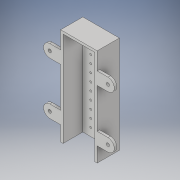
# Autodesk Inventor part: thermometerCover
Saved by Autodesk Inventor 2019.1 (Build 231200000, 200)
## iProperties
Created: 2018-08-04
Part Number: thermometerCover
Material: Generic
Document SubType Name: Modeling
Designer: steele
Density: 1 g/cm^3
Appearance: Default
Author: steele
Autodesk Inventor part; units mm, degrees
ref_plane "YZ Plane" through (0, 0, 0) normal (1, 0, 0) x (0, 1, 0)
ref_plane "XZ Plane" through (0, 0, 0) normal (0, 1, 0) x (-1, 0, 0)
ref_plane "XY Plane" through (0, 0, 0) normal (0, 0, 1) x (1, 0, 0)
sketch "Sketch1" plane through (0, 0, 0) normal (0, 0, 1) x (1, 0, 0)
  line L0 (25.4, -76.2) -> (25.4, 76.2)
  line L1 (25.4, 76.2) -> (-25.4, 76.2)
  line L2 (-25.4, 76.2) -> (-25.4, -76.2)
  line L3 (-25.4, -76.2) -> (25.4, 76.2) construction
  line L4 (25.4, -76.2) -> (-25.4, 76.2) construction
  line L5 (29.3687, -76.2) -> (29.3687, 80.1688)
  line L6 (29.3687, 80.1688) -> (-29.3687, 80.1688)
  line L7 (-29.3687, 80.1688) -> (-29.3687, -76.2)
  line L8 (-29.3687, -80.1688) -> (29.3687, 80.1688) construction
  line L9 (29.3687, -80.1688) -> (-29.3687, 80.1688) construction
  line L10 (-25.4, -76.2) -> (-29.3687, -76.2)
  line L11 (25.4, -76.2) -> (29.3687, -76.2)
  point P0 (0, 0)
  dimension "d2" = 3.9688
  dimension "d3" = 3.9688
  dimension "d5" = 50.8
  dimension "d6" = 152.4
  constraints: 24 end point, 4 midpoint, 2 parallel, 1 point on line
  measures "d2" distance between parallel lines of L5 L0
  measures "d3" distance between parallel lines of L6 L1
  measures "d5" distance between parallel lines of L0 L2
  measures "d6" distance of L0.start L0.end
extrude "Extrusion1" add sketch "Sketch1" along normal blind 31.75
sketch "Sketch2" plane through (0, 0, 0) normal (0, 0, -1) x (-1, 0, 0)
  line L0 (-29.3687, -76.2) -> (-29.3687, 80.1688) projected
  line L1 (29.3687, 80.1688) -> (29.3687, -76.2) projected
  line L2 (-29.3687, 80.1688) -> (29.3687, 80.1688)
  line L3 (29.3687, 80.1688) -> (29.3687, -76.2)
  line L4 (29.3687, -76.2) -> (-29.3687, -76.2)
  line L5 (-29.3687, -76.2) -> (-29.3687, 80.1688)
  point P0 (0, 0)
  constraints: 8 end point, 2 parallel, 1 horizontal, 1 perpendicular
extrude "Extrusion2" add sketch "Sketch2" along normal blind 3.9688
sketch "Sketch5" plane through (0, 0, 31.75) normal (0, 0, 1) x (1, 0, 0)
  line L0 (-29.3687, 80.1688) -> (-29.3687, -76.2)
  line L1 (-29.3687, 42.0688) -> (-46.7574, 42.0688) construction
  line L2 (-29.3687, 31.9088) -> (-46.7574, 31.9088)
  line L3 (-46.7574, 52.2287) -> (-29.3687, 52.2288)
  arc A0 (-46.7574, 52.2287) -> (-46.7574, 31.9088) centre (-46.7574, 42.0688) ccw
  line L4 (29.3687, 80.1688) -> (-29.3687, 80.1688)
  circle A1 centre (-46.7574, 42.0688) radius 2.54
  point P0 (0, 0)
  dimension "d18" = 10.16
  dimension "d21" = 5.08
  constraints: 8 end point, 2 centre point, 2 point on circle, 2 tangent, 1 coincident, 1 parallel, 1 perpendicular, 1 point on line
  measures "d18" radius of A0
  measures "d21" diameter of A1
extrude "Extrusion4" add sketch "Sketch5" against normal blind 3.9688
mirror "Mirror1" about plane through (0, 0, 0) normal (1, 0, 0) of "Extrusion4"
mirror "Mirror2" about plane through (0, 0, 0) normal (0, 1, 0) of "Extrusion4", "Mirror1"
sketch "Sketch6" plane through (0, 0, 0) normal (0, 0, 1) x (1, 0, 0)
  circle A0 centre (-12.7, -63.5) radius 1.5875
  line L0 (-25.4, -76.2) -> (-25.4, 76.2) projected
  line L1 (-25.4, -76.2) -> (25.4, -76.2) construction
  line L2 (-12.7, -63.5) -> (-12.7, 76.2) construction
  line L3 (-25.4, 76.2) -> (25.4, 76.2) construction
  line L4 (-12.7, -63.5) -> (25.4, -63.5) construction
  circle A1 centre (-12.7, -50.8) radius 1.5875
  circle A2 centre (-12.7, -38.1) radius 1.5875
  circle A3 centre (-12.7, -25.4) radius 1.5875
  circle A4 centre (-12.7, -12.7) radius 1.5875
  circle A5 centre (-12.7, 0) radius 1.5875
  circle A6 centre (-12.7, 12.7) radius 1.5875
  circle A7 centre (-12.7, 25.4) radius 1.5875
  circle A8 centre (-12.7, 38.1) radius 1.5875
  circle A9 centre (-12.7, 50.8) radius 1.5875
  circle A10 centre (-12.7, 63.5) radius 1.5875
  circle A11 centre (0, -63.5) radius 1.5875
  circle A12 centre (0, -50.8) radius 1.5875
  circle A13 centre (0, -38.1) radius 1.5875
  circle A14 centre (0, -25.4) radius 1.5875
  circle A15 centre (0, -12.7) radius 1.5875
  circle A16 centre (0, 0) radius 1.5875
  circle A17 centre (0, 12.7) radius 1.5875
  circle A18 centre (0, 25.4) radius 1.5875
  circle A19 centre (0, 38.1) radius 1.5875
  circle A20 centre (0, 50.8) radius 1.5875
  circle A21 centre (0, 63.5) radius 1.5875
  circle A22 centre (12.7, -63.5) radius 1.5875
  circle A23 centre (12.7, -50.8) radius 1.5875
  circle A24 centre (12.7, -38.1) radius 1.5875
  circle A25 centre (12.7, -25.4) radius 1.5875
  circle A26 centre (12.7, -12.7) radius 1.5875
  circle A27 centre (12.7, 0) radius 1.5875
  circle A28 centre (12.7, 12.7) radius 1.5875
  circle A29 centre (12.7, 25.4) radius 1.5875
  circle A30 centre (12.7, 38.1) radius 1.5875
  circle A31 centre (12.7, 50.8) radius 1.5875
  circle A32 centre (12.7, 63.5) radius 1.5875
  dimension "d24" = 3.175
  dimension "d25" = 12.7
  dimension "d26" = 12.7
  dimension "d29" = 12.7
  dimension "d32" = 12.7
  constraints: 33 centre point, 4 end point, 2 horizontal, 2 vertical, 1 point on line, 64 other
  measures "d24" diameter of A0
  measures "d25" distance from line of L0 L2.start
  measures "d26" distance from line of L2.start L1
  measures "d29" distance of L2.start A1.centre
  measures "d32" distance of L2.start A11.centre
extrude "Extrusion5" cut sketch "Sketch6" against normal through all
equation "\"d2\" = wallThickness"
equation "\"d3\" = wallThickness"
equation "\"d5\" = interiorWidth"
equation "\"d6\" = interiorHeight"
equation "\"d7\" = interiorDepth"
equation "\"d9\" = wallThickness"
equation "\"d18\" = tabWidth"
equation "\"d21\" = screwHole"
equation "\"d22\" = wallThickness"
equation "\"interiorWidth\" = 50.8"
equation "\"interiorHeight\" = 152.4"
equation "\"wallThickness\" = 3.96875"
equation "\"interiorDepth\" = 31.75"
equation "\"screwHole\" = 5.08"
equation "\"tabWidth\" = 10.16"
body "Solid1"
